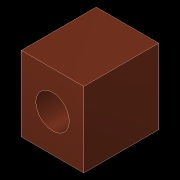
# Autodesk Inventor part: KON_Nietmaschine_Gleitstein
Saved by Autodesk Inventor 2019 (Build 230136000, 136)
## iProperties
Created: 2022-01-03
Part Number: KON_Nietmaschine_Gleitstein
Material: Kupfer
Document SubType Name: Modeling
Designer: Jonas Nebl
Mass: 282.877 g
Surface Area: 83.1943 cm^2
Volume: 31.6418 cm^3
Density: 8.94 g/cm^3
Appearance: Kupfer - satiniert
Author: Jonas Nebl
Autodesk Inventor part; units mm, degrees
ref_plane "YZ Plane" through (0, 0, 0) normal (1, 0, 0) x (0, 1, 0)
ref_plane "XZ Plane" through (0, 0, 0) normal (0, 1, 0) x (-1, 0, 0)
ref_plane "XY Plane" through (0, 0, 0) normal (0, 0, 1) x (1, 0, 0)
sketch "Skizze1" plane through (0, 0, 0) normal (0, 0, 1) x (1, 0, 0)
  line L0 (-15, 18) -> (15, 18)
  line L1 (15, 18) -> (15, -18)
  line L2 (15, -18) -> (-15, -18)
  line L3 (-15, -18) -> (-15, 18)
  circle A0 centre (0, 0) radius 8
  line L4 (-21, 0) -> (21, 0) projected
  line L5 (0, -25.2) -> (0, 25.2) projected
  dimension "d0" = 36
  dimension "d1" = 30
  dimension "d2" = 16
  constraints: 8 end point, 2 parallel, 1 centre point, 1 coincident, 1 horizontal, 1 perpendicular, 1 symmetric about line, 1 other
  measures "d0" distance of L2.end L0.start
  measures "d1" distance of L0.start L0.end
  measures "d2" diameter of A0
extrude "Extrusion1" add sketch "Skizze1" along normal mid plane 36 contours L0 L5 A0 L4 L3 | L0 L1 L4 A0 L5 | L4 A0 L5 L2 L3 | L1 L2 L5 A0 L4
